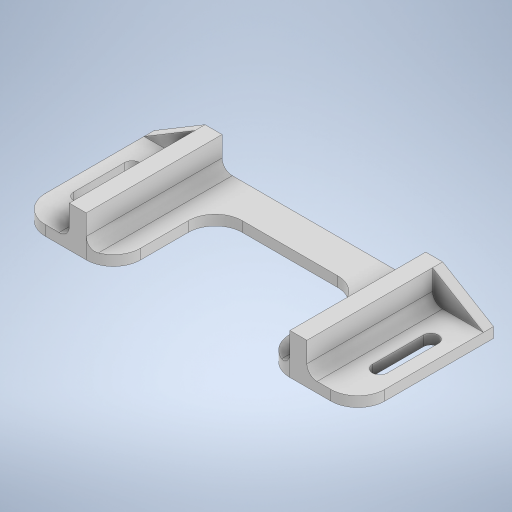
# Autodesk Inventor part: soporte infe sup
Saved by Autodesk Inventor 2024 (Build 280153000, 153)
## iProperties
Created: 2024-04-24
Part Number: soporte infe sup
Material: Generic
Document SubType Name: Modeling
Designer: compu
Density: 1 g/cm^3
Appearance: Default
Author: compu
Autodesk Inventor part; units mm, degrees
ref_plane "YZ Plane" through (0, 0, 0) normal (1, 0, 0) x (0, 1, 0)
ref_plane "XZ Plane" through (0, 0, 0) normal (0, 1, 0) x (-1, 0, 0)
ref_plane "XY Plane" through (0, 0, 0) normal (0, 0, 1) x (1, 0, 0)
sketch "Sketch1" plane through (0, 0, 0) normal (0, 1, 0) x (-1, 0, 0)
  line L0 (72.3196, 0) -> (-72.3196, 0) projected
  line L1 (0, -8.3314) -> (0, 49.9882) projected
  line L2 (50, 0) -> (-50, 0)
  line L3 (-50, 0) -> (-50, 32)
  line L4 (50, 32) -> (50, 0)
  arc A0 (-46.2, 12.5) -> (-41.8, 12.5) centre (-44, 12.5) ccw
  arc A1 (-41.8, 27.5) -> (-46.2, 27.5) centre (-44, 27.5) ccw
  line L5 (-41.8, 12.5) -> (-41.8, 27.5)
  line L6 (-46.2, 12.5) -> (-46.2, 27.5)
  arc A2 (41.8, 12.5) -> (46.2, 12.5) centre (44, 12.5) ccw
  arc A3 (46.2, 27.5) -> (41.8, 27.5) centre (44, 27.5) ccw
  line L7 (41.8, 12.5) -> (41.8, 27.5)
  line L8 (46.2, 12.5) -> (46.2, 27.5)
  arc A4 (50, 32) -> (42, 40) centre (42, 32) ccw
  arc A5 (-42, 40) -> (-50, 32) centre (-42, 32) ccw
  line L9 (-22, 32) -> (-22, 18)
  line L10 (-14, 10) -> (14, 10)
  line L11 (22, 18) -> (22, 32)
  line L12 (-42, 40) -> (-30, 40)
  line L13 (30, 40) -> (42, 40)
  arc A6 (14, 10) -> (22, 18) centre (14, 18) ccw
  arc A7 (30, 40) -> (22, 32) centre (30, 32) ccw
  arc A8 (-22, 32) -> (-30, 40) centre (-30, 32) ccw
  arc A9 (-22, 18) -> (-14, 10) centre (-14, 18) ccw
  point P0 (0, 0)
  point P1 (22, 40)
  point P2 (-22, 10)
  point P3 (-22, 40)
  point P4 (22, 10)
  dimension "d2" = 4.4
  dimension "d3" = 4.4
  dimension "d4" = 15
  dimension "d5" = 0
  dimension "d6" = 12.5
  dimension "d7" = 6
  dimension "d10" = 8
  dimension "d11" = 44
  dimension "d13" = 30
  dimension "d14" = 30
  dimension "d15" = 40
  dimension "d16" = 40
  dimension "d17" = 100
  dimension "d18" = 8
  constraints: 24 end point, 20 point on circle, 17 tangent, 10 centre point, 8 point on line, 6 symmetric about line, 4 equal radius, 4 parallel, 1 collinear, 1 horizontal, 1 perpendicular, 1 vertical, 4 other
  measures "d2" diameter of A0
  measures "d3" diameter of A1
  measures "d4" distance of A1.centre A0.centre
  measures "d5" horizontal distance of A0.centre A1.centre
  measures "d6" distance from line of L2 A0.centre
  measures "d7" distance from line of L3 A0.centre
  measures "d10" radius of A4
  measures "d11" distance of point (22, 10) point (-22, 10)
  measures "d13" distance of point (-22, 40) point (-22, 10)
  measures "d14" distance of point (22, 10) point (22, 40)
  measures "d15" distance between parallel lines of L2 L12
  measures "d16" distance between parallel lines of L13 L2
  measures "d17" distance between parallel lines of L3 L4
  measures "d18" radius of A6
extrude "Extrusion1" add sketch "Sketch1" along normal blind 3
sketch "Sketch2" plane through (0, 3, 0) normal (0, 1, 0) x (1, 0, 0)
  line L0 (-42, -40) -> (-30, -40) projected
  arc A0 (-30, -40) -> (-22, -32) centre (-30, -32) ccw projected
  line L1 (-22, -32) -> (-22, -18) projected
  arc A1 (-14, -10) -> (-22, -18) centre (-14, -18) ccw projected
  line L2 (-14, -10) -> (14, -10) projected
  arc A2 (22, -18) -> (14, -10) centre (14, -18) ccw projected
  line L3 (22, -18) -> (22, -32) projected
  arc A3 (22, -32) -> (30, -40) centre (30, -32) ccw projected
  line L4 (30, -40) -> (42, -40) projected
  arc A4 (42, -40) -> (50, -32) centre (42, -32) ccw projected
  line L5 (50, -32) -> (50, 0) projected
  line L6 (50, 0) -> (-50, 0) projected
  line L7 (-50, 0) -> (-50, -32) projected
  arc A5 (-50, -32) -> (-42, -40) centre (-42, -32) ccw projected
  line L8 (46.2, -12.5) -> (46.2, -27.5) projected
  arc A6 (41.8, -27.5) -> (46.2, -27.5) centre (44, -27.5) ccw projected
  line L9 (41.8, -27.5) -> (41.8, -12.5) projected
  arc A7 (46.2, -12.5) -> (41.8, -12.5) centre (44, -12.5) ccw projected
  line L10 (-41.8, -12.5) -> (-41.8, -27.5) projected
  arc A8 (-46.2, -27.5) -> (-41.8, -27.5) centre (-44, -27.5) ccw projected
  line L11 (-46.2, -27.5) -> (-46.2, -12.5) projected
  arc A9 (-41.8, -12.5) -> (-46.2, -12.5) centre (-44, -12.5) ccw projected
  line L12 (-72.3196, 0) -> (72.3196, 0) projected
  line L13 (0, 8.3314) -> (0, -49.9882) projected
  line L14 (-35, 0) -> (-35, -40)
  line L15 (-42, -40) -> (-30, -40) projected
  line L16 (-30, 0) -> (-30, -40)
  line L17 (50, 0) -> (-50, 0) projected
  line L18 (35, 0) -> (35, -40)
  line L19 (30, 0) -> (30, -40)
  line L20 (30, -40) -> (42, -40) projected
  line L21 (-35, 0) -> (-30, 0)
  line L22 (-35, -40) -> (-30, -40)
  line L23 (30, -40) -> (35, -40)
  line L24 (30, 0) -> (35, 0)
  point P0 (0, 0)
  dimension "d21" = 70
  dimension "d22" = 60
  constraints: 16 end point, 7 point on line, 3 collinear, 3 perpendicular, 2 other
  measures "d21" distance between parallel lines of L18 L14
  measures "d22" distance between parallel lines of L19 L16
extrude "Extrusion2" add sketch "Sketch2" along normal blind 9 contours L14 L6 L16 L0 | L6 L18 L4 L19
sketch "Sketch3" plane through (50, 0, 0) normal (0, 0, -1) x (-1, 0, 0)
  line L0 (0, 0) -> (100, 0) projected
  line L1 (100, 0) -> (100, 3) projected
  line L2 (85, 3) -> (100, 3) projected
  line L3 (85, 3) -> (85, 12) projected
  line L4 (80, 12) -> (85, 12) projected
  line L5 (80, 3) -> (80, 12) projected
  line L6 (20, 3) -> (80, 3) projected
  line L7 (20, 3) -> (20, 12) projected
  line L8 (15, 12) -> (20, 12) projected
  line L9 (15, 3) -> (15, 12) projected
  line L10 (0, 3) -> (15, 3) projected
  line L11 (0, 0) -> (0, 3) projected
  line L12 (85, 12) -> (100, 3)
  line L13 (100, 3) -> (100, 1.5)
  line L14 (100, 0) -> (100, 3) projected
  line L15 (85, 12) -> (82.5, 12)
  line L16 (82.5, 1.5) -> (82.5, 12)
  line L17 (82.5, 1.5) -> (100, 1.5)
  line L18 (15, 12) -> (0, 3)
  line L19 (0, 1.5) -> (17.5, 1.5)
  line L20 (17.5, 1.5) -> (17.5, 12)
  line L21 (15, 12) -> (17.5, 12)
  line L22 (15, 12) -> (20, 12) projected
  line L23 (0, 3) -> (15, 3) projected
  line L24 (0, 3) -> (0, 1.5)
  line L25 (0, 0) -> (0, 3) projected
  point P0 (50, 0)
  constraints: 20 end point, 4 midpoint, 3 perpendicular, 2 collinear, 1 horizontal
extrude "Extrusion3" add sketch "Sketch3" against normal blind 3 contours L11 L10 L9 L8 L20 L19 | L17 L16 L4 L3 L2 L1 | L18 L9 L10 | L2 L3 L12
fillet "Fillet1" radius 3 4 edges at (30, 3, 20) (-35, 3, 21.5) (-30, 3, 20) (35, 3, 21.5)
body "Solid1"
